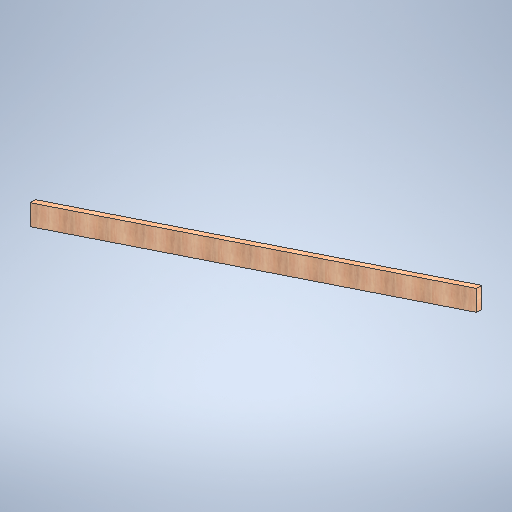
# Autodesk Inventor part: Ceiling_Joist
Saved by Autodesk Inventor 2025 (Build 290162010, 162A)
## iProperties
Created: 2024-09-19
Part Number: Ceiling_Joist
Material: Wood (Birch)
Document SubType Name: Modeling
Designer: Tom
Density: 0.55 g/cm^3
Appearance: Birch - Natural Polished
Author: Tom
Autodesk Inventor part; units mm, degrees
ref_plane "YZ Plane" through (0, 0, 0) normal (1, 0, 0) x (0, 1, 0)
ref_plane "XZ Plane" through (0, 0, 0) normal (0, 1, 0) x (-1, 0, 0)
ref_plane "XY Plane" through (0, 0, 0) normal (0, 0, 1) x (1, 0, 0)
sketch "Sketch1" plane through (0, 0, 0) normal (0, 0, 1) x (1, 0, 0)
  line L0 (0, 0) -> (3175, 1059.3628)
  line L1 (3175, 1059.3628) -> (3175, 1206.6339)
  line L2 (3175, 1206.6339) -> (0, 147.2711)
  line L3 (0, 147.2711) -> (0, 0)
  line L4 (3175, 1059.3628) -> (3263.9, 1089.025)
  line L5 (3263.9, 1089.025) -> (3263.9, 1236.2961)
  line L6 (3263.9, 1236.2961) -> (3175, 1206.6339)
  dimension "d1" = 3175
  dimension "d4" = 139.7
  dimension "d5" = 3263.9
  dimension "d6" = 1089.025
  constraints: 14 end point, 2 collinear, 2 parallel, 2 vertical
  measures "d1" distance between parallel lines of L3 L1
  measures "d4" distance between parallel lines of L2 L0
  measures "d5" horizontal distance of L4.end L0.start
  measures "d6" vertical distance of L4.end L0.start
extrude "Extrusion1" add sketch "Sketch1" along normal blind 38.1 contours L3 L2 L1 L0
body "Solid1"
